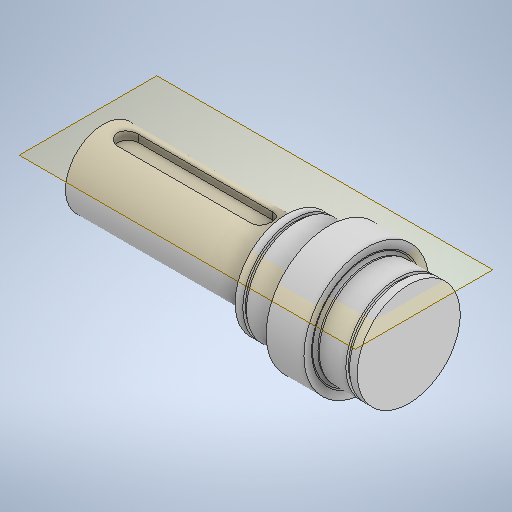
# Autodesk Inventor part: 0
Saved by Autodesk Inventor 2025.3 (Build 293356030, 356C)
## iProperties
Created: 2025-09-24
Part Number: 0
Material: Generisch
Document SubType Name: Modeling
Designer: tobia
Density: 1 g/cm^3
Appearance: Vorgabe
Author: tobia
Autodesk Inventor part; units mm, degrees
ref_plane "YZ Plane" through (0, 0, 0) normal (1, 0, 0) x (0, 1, 0)
ref_plane "XZ Plane" through (0, 0, 0) normal (0, 1, 0) x (-1, 0, 0)
sketch "Skizze1" plane through (0, 0, 0) normal (0, 0, 1) x (1, 0, 0)
  line L0 (0, 0) -> (0, 22)
  line L1 (0, 22) -> (107, 22)
  line L2 (107, 22) -> (107, 30)
  line L3 (107, 30) -> (131.65, 30)
  line L4 (131.65, 30) -> (131.65, 36.5)
  line L5 (131.65, 36.5) -> (153.65, 36.5)
  line L6 (153.65, 36.5) -> (153.65, 30)
  line L7 (153.65, 30) -> (178.3, 30)
  line L8 (178.3, 30) -> (178.3, 0)
  line L9 (178.3, 0) -> (0, 0)
  line L10 (-35.66, 0) -> (213.96, 0) projected
  constraints: 20 end point
revolve "Umdrehung1" add sketch "Skizze1" angle 360 about axis through (-10, 0, 0) along (1, 0, 0)
ref_plane "Arbeitsebene1" through (0, 0, 22) normal (0, 0, 1) x (1, 0, 0)
sketch "Skizze2" plane through (0, 0, 22) normal (0, 0, 1) x (1, 0, 0)
  line L0 (8.5, 0) -> (98.5, 0) construction
  line L1 (14.5, -6) -> (92.5, -6)
  line L2 (92.5, 6) -> (14.5, 6)
  arc A0 (14.5, 6) -> (14.5, -6) centre (14.5, 0) ccw
  arc A1 (92.5, -6) -> (92.5, 6) centre (92.5, 0) ccw
  point P0 (53.5, 0)
  constraints: 8 end point, 6 point on circle, 4 tangent, 2 centre point, 2 point on line, 1 midpoint, 1 parallel
extrude "Extrusion1" cut sketch "Skizze2" against normal blind 5
sketch "Skizze3" plane through (0, 0, 0) normal (0, 0, 1) x (1, 0, 0)
  line L0 (107, 24) -> (107.2, 23.2536)
  line L1 (105.6196, 21.7) -> (104.5, 22)
  line L2 (104.5, 22) -> (104.5, 24)
  line L3 (104.5, 24) -> (107, 24)
  arc A0 (105.6196, 21.7) -> (107.2, 23.2536) centre (106.1294, 22.762) ccw
  line L4 (-35.66, 0) -> (213.96, 0) projected
  constraints: 8 end point, 2 point on circle, 1 centre point
revolve "Umdrehung2" cut sketch "Skizze3" angle 360 about axis through (-10, 0, 0) along (1, 0, 0)
sketch "Skizze4" plane through (0, 0, 0) normal (0, 0, 1) x (1, 0, 0)
  line L0 (111.5, 28.5) -> (113.65, 28.5)
  line L1 (113.65, 28.5) -> (113.65, 30)
  line L2 (113.65, 30) -> (111.5, 30)
  line L3 (111.5, 30) -> (111.5, 28.5)
  line L4 (-35.66, 0) -> (213.96, 0) projected
  constraints: 8 end point, 2 parallel, 1 horizontal, 1 perpendicular
revolve "Umdrehung3" cut sketch "Skizze4" angle 360 about axis through (-10, 0, 0) along (1, 0, 0)
sketch "Skizze5" plane through (0, 0, 0) normal (0, 0, 1) x (1, 0, 0)
  line L0 (131.65, 32) -> (131.85, 31.2536)
  line L1 (130.2696, 29.7) -> (129.15, 30)
  line L2 (129.15, 30) -> (129.15, 32)
  line L3 (129.15, 32) -> (131.65, 32)
  arc A0 (130.2696, 29.7) -> (131.85, 31.2536) centre (130.7794, 30.762) ccw
  line L4 (-35.66, 0) -> (213.96, 0) projected
  constraints: 8 end point, 2 point on circle, 1 centre point
revolve "Umdrehung4" cut sketch "Skizze5" angle 360 about axis through (-10, 0, 0) along (1, 0, 0)
sketch "Skizze6" plane through (0, 0, 0) normal (0, 0, 1) x (1, 0, 0)
  line L0 (173.8, 28.5) -> (171.65, 28.5)
  line L1 (171.65, 28.5) -> (171.65, 30)
  line L2 (171.65, 30) -> (173.8, 30)
  line L3 (173.8, 30) -> (173.8, 28.5)
  line L4 (-35.66, 0) -> (213.96, 0) projected
  constraints: 8 end point, 2 parallel, 1 horizontal, 1 perpendicular
revolve "Umdrehung5" cut sketch "Skizze6" angle 360 about axis through (-10, 0, 0) along (1, 0, 0)
sketch "Skizze7" plane through (0, 0, 0) normal (0, 0, 1) x (1, 0, 0)
  line L0 (153.65, 32) -> (153.45, 31.2536)
  line L1 (155.0304, 29.7) -> (156.15, 30)
  line L2 (156.15, 30) -> (156.15, 32)
  line L3 (156.15, 32) -> (153.65, 32)
  arc A0 (153.45, 31.2536) -> (155.0304, 29.7) centre (154.5206, 30.762) ccw
  line L4 (-35.66, 0) -> (213.96, 0) projected
  constraints: 8 end point, 2 point on circle, 1 centre point
revolve "Umdrehung6" cut sketch "Skizze7" angle 360 about axis through (-10, 0, 0) along (1, 0, 0)
